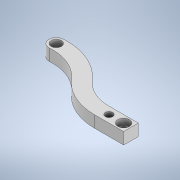
# Autodesk Inventor part: huzo1
Saved by Autodesk Inventor 2020 (Build 240168000, 168)
## iProperties
Created: 2019-08-09
Part Number: huzo1
Material: Generic
Document SubType Name: Modeling
Designer: Horváth Patrik
Density: 1 g/cm^3
Appearance: Default
Author: Horváth Patrik
Autodesk Inventor part; units mm, degrees
ref_plane "YZ Plane" through (0, 0, 0) normal (1, 0, 0) x (0, 1, 0)
ref_plane "XZ Plane" through (0, 0, 0) normal (0, 1, 0) x (-1, 0, 0)
ref_plane "XY Plane" through (0, 0, 0) normal (0, 0, 1) x (1, 0, 0)
sketch "Sketch1" plane through (0, 0, 0) normal (0, 0, 1) x (1, 0, 0)
  line L0 (-7, 0) -> (7, 0) construction
  line L1 (0, -2.8) -> (0, 2.8) construction
  line L2 (5, -2) -> (-5, -2)
  line L3 (-5, -2) -> (-5, 2)
  line L4 (-5, 2) -> (5, 2)
  line L5 (5, 2) -> (5, -2)
  line L6 (5, -2) -> (-5, 2) construction
  line L7 (-5, -2) -> (5, 2) construction
  point P0 (0, 0)
  dimension "d8" = 4
  dimension "d9" = 10
  constraints: 12 end point, 2 midpoint, 2 parallel, 1 horizontal, 1 perpendicular
  measures "d8" distance of L2.end L3.end
  measures "d9" distance between parallel lines of L5 L3
extrude "Extrusion1" add sketch "Sketch1" along normal blind 5
sketch "Sketch2" plane through (-5, 2, 0) normal (0, 1, 0) x (1, 0, 0)
  line L0 (10, 0) -> (10, -5) projected
  line L1 (10, 0) -> (0, 0) projected
  point P0 (5, 0)
  point P1 (7.5, -2.5)
  point P2 (10, -2.5)
  dimension "d12" = 2.5
  constraints: 1 horizontal alignment, 1 midpoint
  measures "d12" distance from line of L0 point (7.5, -2.5)
hole "Hole1" at (2.5, 2, 2.5) direction (0, -1, 0) diameter 2.5 depth 10 tip angle 118 counterbore diameter 4 counterbore depth 2
sketch "Sketch3" plane through (-5, -2, 0) normal (0, -1, 0) x (1, 0, 0)
  circle A0 centre (7.5, 2.5) radius 1.25 projected
  point P0 (5, 0)
  point P1 (2.5, 2.5)
  dimension "d21" = 5
  constraints: 1 horizontal alignment
  measures "d21" distance of A0.centre point (2.5, 2.5)
hole "Hole2" at (-2.5, -2, 2.5) direction (0, 1, 0) diameter 2.5 depth 10 tip angle 118 counterbore diameter 4 counterbore depth 2
sketch "Sketch4" plane through (-5, 2, 0) normal (0, 1, 0) x (1, 0, 0)
  line L0 (0, 0) -> (0, -5) projected
  arc A0 (-12.5, 3.2297) -> (0, -2.5) centre (0, 14) ccw construction
  arc A1 (-14.3939, 1.5978) -> (0, -5) centre (0, 14) ccw
  arc A2 (-10.6061, 4.8615) -> (0, 0) centre (0, 14) ccw
  arc A3 (-10.6061, 4.8615) -> (-14.3939, 1.5978) centre (-12.5, 3.2297) ccw construction
  line L1 (10, 0) -> (0, 0) projected
  line L2 (10, -5) -> (0, -5) projected
  arc A4 (-12.5, 3.2297) -> (-27.5, 9.5) centre (-26.2704, -8.6352) ccw construction
  arc A5 (-10.6061, 4.8615) -> (-27.6691, 11.9943) centre (-26.2704, -8.6352) ccw
  arc A6 (-14.3939, 1.5978) -> (-27.3309, 7.0057) centre (-26.2704, -8.6352) ccw
  arc A7 (-14.3939, 1.5978) -> (-10.6061, 4.8615) centre (-12.5, 3.2297) ccw construction
  arc A8 (-27.6691, 11.9943) -> (-27.3309, 7.0057) centre (-27.5, 9.5) ccw
  circle A9 centre (2.5, -2.5) radius 1.25 projected
  circle A10 centre (-27.5, 9.5) radius 1.75
  point P0 (5, 0)
  point P1 (0, 0)
  point P2 (-14.3939, 1.5978)
  point P3 (0, -5)
  dimension "d30" = 15
  dimension "d31" = 15
  dimension "d32" = 12
  dimension "d33" = 14
  dimension "d34" = 3.5
  constraints: 18 point on circle, 10 centre point, 10 tangent, 1 coincident, 1 midpoint
  measures "d30" horizontal distance of A4.end A0.start
  measures "d31" horizontal distance of A4.start A9.centre
  measures "d32" vertical distance of A9.centre A4.end
  measures "d33" radius of A2
  measures "d34" diameter of A10
extrude "Extrusion2" add sketch "Sketch4" against normal blind 4 contours L0 A1 A6 A8 A5 A2
body "Solid1"
